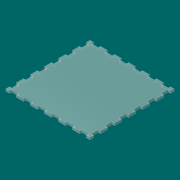
# Autodesk Inventor part: topBottomPanel
Saved by Autodesk Inventor 2016 (Build 200138000, 138)
## iProperties
Created: 2015-10-05
Part Number: topBottomPanel
Material: Polycarbonate, Clear
Document SubType Name: Modeling
Designer: sawai
Density: 1.2 g/cm^3
Appearance: Polycarbonate - Clear
Author: sawai
Autodesk Inventor part; units mm, degrees
ref_plane "YZ Plane" through (0, 0, 0) normal (1, 0, 0) x (0, 1, 0)
ref_plane "XZ Plane" through (0, 0, 0) normal (0, 1, 0) x (-1, 0, 0)
ref_plane "XY Plane" through (0, 0, 0) normal (0, 0, 1) x (1, 0, 0)
sketch "Sketch1" plane through (0, 0, 0) normal (0, 0, 1) x (1, 0, 0)
  line L0 (-60, -60) -> (60, -60)
  line L1 (60, -60) -> (60, 60)
  line L2 (60, 60) -> (-60, 60)
  line L3 (-60, 60) -> (-60, -60)
  line L4 (-60, -60) -> (60, 60) construction
  line L5 (60, -60) -> (-60, 60) construction
  point P0 (0, 0)
  dimension "d0" = 120
  dimension "d1" = 120
  constraints: 12 end point, 2 midpoint, 2 parallel, 1 horizontal, 1 perpendicular
  measures "d0" distance of L2.end L1.end
  measures "d1" distance of L1.end L0.end
extrude "Extrusion1" add sketch "Sketch1" along normal blind 3.175
sketch "Sketch5" plane through (0, 0, 3.175) normal (0, 0, 1) x (1, 0, 0)
  line L0 (-60, -60) -> (60, -60) projected
  line L1 (60, -60) -> (60, 60) projected
  line L2 (60, 60) -> (-60, 60) projected
  line L3 (-60, 60) -> (-60, -60) projected
  line L4 (-60, -60) -> (60, -60) projected
  line L5 (55, -60) -> (45, -60)
  line L6 (45, -60) -> (45, -56.825)
  line L7 (45, -56.825) -> (55, -56.825)
  line L8 (55, -56.825) -> (55, -60)
  point P0 (0, 0)
  dimension "d25" = 10
  dimension "d27" = 5
  dimension "d41" = 3.175
  constraints: 8 end point, 2 parallel, 1 horizontal, 1 perpendicular, 1 point on line
  measures "d25" distance of L6.end L7.end
  measures "d27" distance between parallel lines of L1 L8
  measures "d41" distance between parallel lines of L0 L7
extrude "Extrusion3" cut sketch "Sketch5" against normal up to surface (3.175 mm away) contours L6 L7 L8 L0
pattern_linear "Rectangular Pattern2" count 6 spacing 20 along (-1, 0, 0) of "Extrusion3"
mirror "Mirror2" about plane through (0, 0, 0) normal (0, 1, 0) of "Extrusion3", "Rectangular Pattern2"
sketch "Sketch6" plane through (0, 0, 3.175) normal (0, 0, 1) x (1, 0, 0)
  line L0 (-60, -60) -> (-55, -60) projected
  line L1 (-45, -60) -> (-35, -60) projected
  line L2 (-25, -60) -> (-15, -60) projected
  line L3 (-5, -60) -> (5, -60) projected
  line L4 (15, -60) -> (25, -60) projected
  line L5 (35, -60) -> (45, -60) projected
  line L6 (60, -60) -> (60, 60) projected
  line L7 (60, 60) -> (55, 60) projected
  line L8 (45, 60) -> (35, 60) projected
  line L9 (25, 60) -> (15, 60) projected
  line L10 (5, 60) -> (-5, 60) projected
  line L11 (-15, 60) -> (-25, 60) projected
  line L12 (-35, 60) -> (-45, 60) projected
  line L13 (-60, 60) -> (-60, -60) projected
  line L14 (-60, -55) -> (-56.825, -55)
  line L15 (-56.825, -55) -> (-56.825, -45)
  line L16 (-56.825, -45) -> (-60, -45)
  line L17 (-60, -45) -> (-60, -55)
  line L18 (55, -60) -> (60, -60) projected
  line L19 (-55, 60) -> (-60, 60) projected
  line L20 (-55, 56.825) -> (-55, 60) projected
  line L21 (-55, -60) -> (-55, -56.825) projected
  line L22 (-55, -56.825) -> (-45, -56.825) projected
  line L23 (-45, -56.825) -> (-45, -60) projected
  line L24 (-35, -60) -> (-35, -56.825) projected
  line L25 (-35, -56.825) -> (-25, -56.825) projected
  line L26 (-25, -56.825) -> (-25, -60) projected
  line L27 (-15, -60) -> (-15, -56.825) projected
  line L28 (-15, -56.825) -> (-5, -56.825) projected
  line L29 (-5, -56.825) -> (-5, -60) projected
  line L30 (5, -60) -> (5, -56.825) projected
  line L31 (5, -56.825) -> (15, -56.825) projected
  line L32 (15, -56.825) -> (15, -60) projected
  line L33 (25, -60) -> (25, -56.825) projected
  line L34 (25, -56.825) -> (35, -56.825) projected
  line L35 (35, -56.825) -> (35, -60) projected
  line L36 (45, -60) -> (45, -56.825) projected
  line L37 (45, -56.825) -> (55, -56.825) projected
  line L38 (55, -56.825) -> (55, -60) projected
  line L39 (55, 60) -> (55, 56.825) projected
  line L40 (55, 56.825) -> (45, 56.825) projected
  line L41 (45, 56.825) -> (45, 60) projected
  line L42 (35, 60) -> (35, 56.825) projected
  line L43 (35, 56.825) -> (25, 56.825) projected
  line L44 (25, 56.825) -> (25, 60) projected
  line L45 (15, 60) -> (15, 56.825) projected
  line L46 (15, 56.825) -> (5, 56.825) projected
  line L47 (5, 56.825) -> (5, 60) projected
  line L48 (-5, 60) -> (-5, 56.825) projected
  line L49 (-5, 56.825) -> (-15, 56.825) projected
  line L50 (-15, 56.825) -> (-15, 60) projected
  line L51 (-25, 60) -> (-25, 56.825) projected
  line L52 (-25, 56.825) -> (-35, 56.825) projected
  line L53 (-35, 56.825) -> (-35, 60) projected
  line L54 (-45, 60) -> (-45, 56.825) projected
  line L55 (-45, 56.825) -> (-55, 56.825) projected
  point P0 (0, 0)
  dimension "d34" = 10
  dimension "d35" = 5
  dimension "d42" = 3.175
  constraints: 8 end point, 2 parallel, 1 horizontal, 1 perpendicular, 1 point on line
  measures "d34" distance of L14.end L15.end
  measures "d35" distance between parallel lines of L0 L14
  measures "d42" distance between parallel lines of L13 L15
extrude "Extrusion4" cut sketch "Sketch6" against normal up to surface (3.175 mm away) contours L13 L16 L15 L14
pattern_linear "Rectangular Pattern3" count 6 spacing 20 along (0, 1, 0) of "Extrusion4"
mirror "Mirror3" about plane through (0, 0, 0) normal (1, 0, 0) of "Extrusion4", "Rectangular Pattern3"
equation "\"d0\" = width"
equation "\"d1\" = depth"
equation "\"d2\" = materialThickness"
equation "\"d25\" = notchWidth"
equation "\"d27\" = 0 * materialThickness + 0.5 * width - 5.5 * notchWidth"
equation "\"d41\" = materialThickness"
equation "\"d32\" = 2 * notchWidth"
equation "\"d34\" = notchWidth"
equation "\"d35\" = 0 * materialThickness + 0.5 * depth - 5.5 * notchWidth"
equation "\"d42\" = materialThickness"
equation "\"d40\" = 2 * notchWidth"
equation "\"width\" = 120"
equation "\"depth\" = 120"
equation "\"materialThickness\" = 3.175"
equation "\"laserKerf\" = 0.1"
equation "\"cardPinDiameter\" = 3"
equation "\"cardFillet\" = 2.88"
equation "\"cardSelected\" = 1"
equation "\"cardThickness\" = 0.76"
equation "\"cardHeight\" = 53.98"
equation "\"cardWidth\" = 85.6"
equation "\"centeralShaftDiameter\" = 8"
equation "\"cardClearence\" = 0.5"
equation "\"bearingOd\" = 22"
equation "\"bearingWidth\" = 8"
equation "\"axleHeight\" = 95"
equation "\"nutTrapDepth\" = 2.5"
equation "\"nutTrapwidth\" = 5.5"
equation "\"nutTrapClearence\" = 2"
equation "\"magnetLength\" = 3"
equation "\"magnetDiameter\" = 6"
equation "\"magnetProtusion\" = 0.25"
equation "\"notchWidth\" = 10"
equation "\"spoolThickness\" = 5.588"
body "Solid1"
